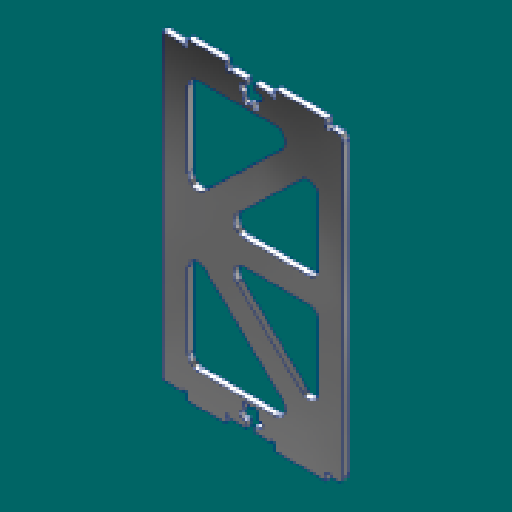
# Autodesk Inventor part: IntakeRamp
Saved by Autodesk Inventor 2023.1 (Build 271208000, 208)
## iProperties
Created: 2022-11-11
Part Number: IntakeRamp
Material: Aluminum 6061
Document SubType Name: Modeling
Designer: zac-h
Density: 2.7 g/cm^3
Appearance: Aluminum - Flat
Mass: 67.9744 g
Surface Area: 202.14 cm^2
Volume: 25.1757 cm^3
Author: zac-h
Autodesk Inventor part; units mm, degrees
ref_plane "YZ Plane" through (0, 0, 0) normal (1, 0, 0) x (0, 1, 0)
ref_plane "XZ Plane" through (0, 0, 0) normal (0, 1, 0) x (-1, 0, 0)
ref_plane "XY Plane" through (0, 0, 0) normal (0, 0, 1) x (1, 0, 0)
sketch "Sketch1" plane through (0, 0, 0) normal (0, 0, 1) x (1, 0, 0)
  line L0 (0, 0) -> (19.05, 0) projected
  line L1 (19.05, 0) -> (19.05, 3) projected
  line L2 (0, 3) -> (19.05, 3) construction
  line L3 (0, 0) -> (0, 3) projected
  line L4 (29.591, 3) -> (33.909, 3) construction
  line L5 (44.45, 0) -> (69.85, 0) projected
  line L6 (69.85, 0) -> (69.85, 3) projected
  line L7 (44.45, 3) -> (69.85, 3) construction
  line L8 (44.45, 0) -> (44.45, 3) projected
  line L9 (0, 3) -> (-6.35, 3)
  line L10 (0, 3) -> (6.35, 3) construction
  line L11 (-6.35, 3) -> (-6.35, 79.2)
  line L12 (-6.35, 79.2) -> (78.74, 79.2)
  line L13 (69.85, 3) -> (78.74, 3)
  line L14 (78.74, 3) -> (78.74, 79.2)
  line L15 (19.05, 3) -> (29.591, 3)
  line L16 (44.45, 3) -> (33.909, 3)
  line L17 (33.909, 3) -> (33.909, 6)
  line L18 (33.909, 6) -> (35.814, 6)
  line L19 (35.814, 6) -> (35.814, 12.35)
  line L20 (35.814, 12.35) -> (27.686, 12.35)
  line L21 (27.686, 12.35) -> (27.686, 6)
  line L22 (27.686, 6) -> (29.591, 6)
  line L23 (29.591, 6) -> (29.591, 3)
  circle A0 centre (20.3, 3) radius 1.25
  circle A1 centre (-1.25, 3) radius 1.25
  circle A2 centre (43.2, 3) radius 1.25
  circle A3 centre (71.1, 3) radius 1.25
  circle A4 centre (35.814, 7.75) radius 1.75
  circle A5 centre (27.686, 7.75) radius 1.75
  circle A6 centre (34.064, 12.35) radius 1.75
  circle A7 centre (29.436, 12.35) radius 1.75
  point P0 (28.6385, 6)
  point P1 (21.55, 3)
  point P2 (27.686, 9.5)
  point P3 (31.186, 12.35)
  point P4 (32.314, 12.35)
  point P5 (35.814, 9.5)
  point P6 (41.95, 3)
  point P7 (72.35, 3)
  point P8 (-2.5, 3)
  dimension "d9" = 2.5
  dimension "d10" = 3.5
  dimension "d11" = 3.5
  dimension "d0" = 6.35
  dimension "d1" = 180
  dimension "d2" = 76.2
  dimension "d3" = 8.89
  dimension "d4" = 3
  dimension "d5" = 8.128
  dimension "d6" = 6.35
  constraints: 30 end point, 10 point on line, 6 perpendicular, 5 horizontal, 3 collinear, 2 vertical, 1 midpoint, 1 parallel, 24 other
  measures "d0" distance of L2.start L9.end
  measures "d1" angle of L9 L10
  measures "d2" distance of L9.end L11.end
  measures "d3" distance of L6.end L13.end
  measures "d4" distance of L4.end L17.end
  measures "d5" distance between parallel lines of L19 L21
  measures "d6" distance from line of point (28.638, 6) L20
extrude "Extrusion1" add sketch "Sketch1" along normal blind 3 contours L3 A1 L9 L11 L12 L14 L13 A3 L6 L5 L8 A2 L16 L17 L18 A4 L19 A6 L20 A7 L21 A5 L22 L23 L15 A0 L1 L0
fillet "Fillet1" radius 1.75 2 edges at (31.186, 12.35, 1.5) (32.314, 12.35, 1.5)
mirror "Mirror1" about plane through (78.74, 79.2, 0) normal (0, 1, 0) of "Extrusion1"
sketch "Sketch2" plane through (0, 0, 3) normal (0, 0, 1) x (1, 0, 0)
  arc A0 (30.593, 13.663) -> (32.907, 13.663) centre (31.75, 14.9759) ccw projected
  arc A1 (35.814, 12.35) -> (32.907, 13.663) centre (34.064, 12.35) ccw projected
  line L0 (35.814, 12.35) -> (35.814, 9.5) projected
  arc A2 (35.814, 6) -> (35.814, 9.5) centre (35.814, 7.75) ccw projected
  line L1 (35.814, 6) -> (33.909, 6) projected
  line L2 (33.909, 6) -> (33.909, 3) projected
  line L3 (33.909, 3) -> (41.95, 3) projected
  arc A3 (44.45, 3) -> (41.95, 3) centre (43.2, 3) ccw projected
  line L4 (44.45, 3) -> (44.45, 0) projected
  line L5 (44.45, 0) -> (69.85, 0) projected
  line L6 (69.85, 0) -> (69.85, 3) projected
  arc A4 (72.35, 3) -> (69.85, 3) centre (71.1, 3) ccw projected
  line L7 (72.35, 3) -> (78.74, 3) projected
  line L8 (78.74, 3) -> (78.74, 155.4) projected
  line L9 (72.35, 155.4) -> (78.74, 155.4) projected
  arc A5 (69.85, 155.4) -> (72.35, 155.4) centre (71.1, 155.4) ccw projected
  line L10 (69.85, 158.4) -> (69.85, 155.4) projected
  line L11 (44.45, 158.4) -> (69.85, 158.4) projected
  line L12 (44.45, 155.4) -> (44.45, 158.4) projected
  arc A6 (41.95, 155.4) -> (44.45, 155.4) centre (43.2, 155.4) ccw projected
  line L13 (33.909, 155.4) -> (41.95, 155.4) projected
  line L14 (33.909, 152.4) -> (33.909, 155.4) projected
  line L15 (35.814, 152.4) -> (33.909, 152.4) projected
  arc A7 (35.814, 148.9) -> (35.814, 152.4) centre (35.814, 150.65) ccw projected
  line L16 (35.814, 146.05) -> (35.814, 148.9) projected
  arc A8 (32.314, 146.05) -> (35.814, 146.05) centre (34.064, 146.05) ccw projected
  line L17 (31.186, 146.05) -> (32.314, 146.05) projected
  arc A9 (27.686, 146.05) -> (31.186, 146.05) centre (29.436, 146.05) ccw projected
  line L18 (27.686, 148.9) -> (27.686, 146.05) projected
  arc A10 (27.686, 152.4) -> (27.686, 148.9) centre (27.686, 150.65) ccw projected
  line L19 (29.591, 152.4) -> (27.686, 152.4) projected
  line L20 (29.591, 155.4) -> (29.591, 152.4) projected
  line L21 (21.55, 155.4) -> (29.591, 155.4) projected
  arc A11 (19.05, 155.4) -> (21.55, 155.4) centre (20.3, 155.4) ccw projected
  line L22 (19.05, 158.4) -> (19.05, 155.4) projected
  line L23 (0, 158.4) -> (19.05, 158.4) projected
  line L24 (0, 155.4) -> (0, 158.4) projected
  arc A12 (-2.5, 155.4) -> (0, 155.4) centre (-1.25, 155.4) ccw projected
  line L25 (-6.35, 155.4) -> (-2.5, 155.4) projected
  line L26 (-6.35, 3) -> (-6.35, 155.4) projected
  line L27 (-6.35, 3) -> (-2.5, 3) projected
  arc A13 (0, 3) -> (-2.5, 3) centre (-1.25, 3) ccw projected
  line L28 (0, 3) -> (0, 0) projected
  line L29 (0, 0) -> (19.05, 0) projected
  line L30 (19.05, 0) -> (19.05, 3) projected
  arc A14 (21.55, 3) -> (19.05, 3) centre (20.3, 3) ccw projected
  line L31 (21.55, 3) -> (29.591, 3) projected
  line L32 (29.591, 3) -> (29.591, 6) projected
  line L33 (29.591, 6) -> (27.686, 6) projected
  arc A15 (27.686, 9.5) -> (27.686, 6) centre (27.686, 7.75) ccw projected
  line L34 (27.686, 9.5) -> (27.686, 12.35) projected
  arc A16 (30.593, 13.663) -> (27.686, 12.35) centre (29.436, 12.35) ccw projected
  line L35 (6.35, 15.7) -> (66.04, 15.7)
  line L36 (66.04, 15.7) -> (66.04, 142.7)
  line L37 (66.04, 142.7) -> (6.35, 142.7)
  line L38 (6.35, 142.7) -> (6.35, 15.7)
  line L39 (6.35, 79.2) -> (66.04, 79.2) construction
  line L40 (6.35, 72.85) -> (66.04, 72.85)
  line L41 (66.04, 85.55) -> (6.35, 85.55)
  arc A17 (6.35, 85.55) -> (6.35, 72.85) centre (6.35, 79.2) ccw
  arc A18 (66.04, 72.85) -> (66.04, 85.55) centre (66.04, 79.2) ccw
  line L42 (66.04, 142.7) -> (6.35, 79.2) construction
  line L43 (61.4132, 147.0492) -> (1.7232, 83.5492)
  line L44 (10.9768, 74.8508) -> (70.6668, 138.3508)
  arc A19 (70.6668, 138.3508) -> (61.4132, 147.0492) centre (66.04, 142.7) ccw
  arc A20 (1.7232, 83.5492) -> (10.9768, 74.8508) centre (6.35, 79.2) ccw
  line L45 (66.04, 15.7) -> (6.35, 79.2) construction
  line L46 (70.6668, 20.0492) -> (10.9768, 83.5492)
  line L47 (1.7232, 74.8508) -> (61.4132, 11.3508)
  arc A21 (61.4132, 11.3508) -> (70.6668, 20.0492) centre (66.04, 15.7) ccw
  arc A22 (10.9768, 83.5492) -> (1.7232, 74.8508) centre (6.35, 79.2) ccw
  point P0 (36.195, 79.2)
  point P1 (36.195, 110.95)
  point P2 (36.195, 47.45)
  point P3 (57.325, 15.7)
  point P4 (6.35, 69.9287)
  point P5 (21.034, 72.85)
  point P6 (66.04, 24.9713)
  point P7 (66.04, 133.4287)
  point P8 (21.034, 85.55)
  point P9 (6.35, 88.4713)
  point P10 (57.325, 142.7)
  dimension "d13" = 12.7
  dimension "d14" = 12.7
  dimension "d15" = 12.7
  dimension "d16" = 12.7
  dimension "d28" = 12.7
  dimension "d29" = 12.7
  constraints: 32 end point, 12 point on circle, 12 tangent, 6 centre point, 5 midpoint, 5 parallel, 1 concentric, 1 horizontal, 1 perpendicular
  measures "d13" distance between parallel lines of L26 L38
  measures "d14" distance between parallel lines of L36 L8
  measures "d15" distance between parallel lines of L9 L37
  measures "d16" distance between parallel lines of L7 L35
  measures "d28" diameter of A18
  measures "d29" diameter of A20
extrude "Extrusion2" cut sketch "Sketch2" against normal blind 3 contours L38 L47 L35 | L46 L40 L36 | L38 L37 L43 | L44 L36 L41
fillet "Fillet2" radius 3.175 2 edges at (78.74, 155.4, 1.5) (78.74, 3, 1.5)
fillet "Fillet3" radius 5 12 edges at (21.034, 72.85, 1.5) (66.04, 72.85, 1.5) (66.04, 24.9713, 1.5) (66.04, 133.4287, 1.5) (66.04, 85.55, 1.5) (21.034, 85.55, 1.5) (57.325, 15.7, 1.5) (6.35, 15.7, 1.5) (6.35, 69.9287, 1.5) (6.35, 88.4713, 1.5) (6.35, 142.7, 1.5) (57.325, 142.7, 1.5)
body "Solid1"
